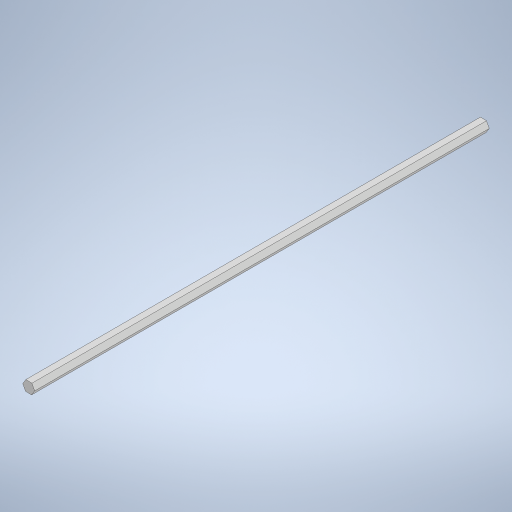
# Autodesk Inventor part: 4-bar intake (22) shaft
Saved by Autodesk Inventor 2023 (Build 270158030, 158C)
## iProperties
Created: 2022-07-18
Part Number: 4-bar intake (22) shaft
Material: Generic
Document SubType Name: Modeling
Designer: kt1040502
Density: 1 g/cm^3
Appearance: Default
Author: kt1040502
Autodesk Inventor part; units mm, degrees
ref_plane "YZ Plane" through (0, 0, 0) normal (1, 0, 0) x (0, 1, 0)
ref_plane "XZ Plane" through (0, 0, 0) normal (0, 1, 0) x (-1, 0, 0)
ref_plane "XY Plane" through (0, 0, 0) normal (0, 0, 1) x (1, 0, 0)
sketch "Sketch3" plane through (0, 0, 0) normal (0, 0, 1) x (1, 0, 0)
  circle A0 centre (0, 0) radius 6.35
  line L0 (7.3277, -0.2611) -> (3.4378, -6.4765)
  line L1 (3.4378, -6.4765) -> (-3.8899, -6.2154)
  line L2 (-3.8899, -6.2154) -> (-7.3277, 0.2611)
  line L3 (-7.3277, 0.2611) -> (-3.4378, 6.4765)
  line L4 (-3.4378, 6.4765) -> (3.8899, 6.2154)
  line L5 (3.8899, 6.2154) -> (7.3277, -0.2611)
  point P0 (5.6088, 2.9772)
  dimension "d5" = 12.7
  constraints: 12 end point, 2 coincident, 1 midpoint, 16 other
extrude "Extrusion3" add sketch "Sketch3" along normal blind 558.8
body "Solid2"
